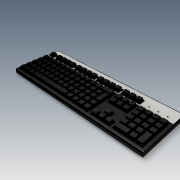
# Autodesk Inventor part: Teclado HP
Saved by Autodesk Inventor 2017 SP1 (Build 210196100, 196)
## iProperties
Created: 2013-08-30
Part Number: Teclado HP
Material: Generic
Document SubType Name: Modeling
Designer: MARCELO
Density: 1 g/cm^3
Mass: 1343.46 g
Surface Area: 2506.42 cm^2
Volume: 1343.46 cm^3
Appearance: Low Gloss - Black
Author: MARCELO
Autodesk Inventor part; units mm, degrees
ref_plane "YZ Plane" through (0, 0, 0) normal (1, 0, 0) x (0, 1, 0)
ref_plane "XZ Plane" through (0, 0, 0) normal (0, 1, 0) x (-1, 0, 0)
ref_plane "XY Plane" through (0, 0, 0) normal (0, 0, 1) x (1, 0, 0)
sketch "Sketch1" plane through (0, 0, 0) normal (0, 1, 0) x (-1, 0, 0)
  line L0 (0, 0) -> (-450, 0)
  line L1 (-450, 0) -> (-450, -160)
  line L2 (-450, -160) -> (0, -160)
  line L3 (0, -160) -> (0, 0)
  dimension "d0" = 450
  dimension "d2" = 160
  constraints: 8 end point, 2 parallel, 1 horizontal, 1 perpendicular
  measures "d0" distance between parallel lines of L1 L3
  measures "d2" distance between parallel lines of L2 L0
extrude "Extrusion1" add sketch "Sketch1" along normal blind 17
fillet "Fillet1" radius 10 2 edges at (450, 8.5, -160) (0, 8.5, -160)
fillet "Fillet1" radius 5 2 edges at (225, 17, 0) (225, 0, 0)
sketch "Sketch2" plane through (0, 17, 0) normal (0, 1, 0) x (1, 0, 0)
  line L0 (450, 5) -> (0, 5) projected
  line L1 (450, 5) -> (450, 150) projected
  line L2 (0, 150) -> (0, 5) projected
  line L3 (6, 9) -> (288, 9)
  line L4 (288, 111) -> (6, 111)
  line L5 (6, 111) -> (6, 9)
  line L6 (293, 31) -> (313, 31)
  line L7 (313, 31) -> (313, 51)
  line L8 (313, 51) -> (335, 51)
  line L9 (335, 51) -> (335, 31)
  line L10 (335, 31) -> (355, 31)
  line L11 (355, 31) -> (355, 9)
  line L12 (355, 9) -> (293, 9)
  line L13 (360, 9) -> (442, 9)
  line L14 (442, 9) -> (442, 111)
  line L15 (442, 111) -> (360, 111)
  line L16 (360, 111) -> (360, 9)
  line L17 (6, 117) -> (28, 117)
  line L18 (28, 117) -> (28, 139)
  line L19 (28, 139) -> (6, 139)
  line L20 (6, 139) -> (6, 117)
  line L21 (289, 117) -> (207, 117)
  line L22 (207, 117) -> (207, 139)
  line L23 (207, 139) -> (289, 139)
  line L24 (289, 139) -> (289, 117)
  line L25 (203, 117) -> (121, 117)
  line L26 (121, 117) -> (121, 139)
  line L27 (121, 139) -> (203, 139)
  line L28 (203, 139) -> (203, 117)
  line L29 (35, 139) -> (117, 139)
  line L30 (117, 139) -> (117, 117)
  line L31 (117, 117) -> (35, 117)
  line L32 (35, 117) -> (35, 139)
  line L33 (293, 111) -> (355, 111)
  line L34 (355, 111) -> (355, 69)
  line L35 (355, 69) -> (293, 69)
  line L36 (293, 117) -> (355, 117)
  line L37 (355, 117) -> (355, 139)
  line L38 (355, 139) -> (293, 139)
  line L39 (293, 139) -> (293, 117)
  circle A0 centre (376, 126) radius 2
  circle A1 centre (401, 126) radius 2
  circle A2 centre (426, 126) radius 2
  line L40 (401, 126) -> (401, 111) construction
  line L41 (288, 111) -> (288, 9)
  line L42 (440, 160) -> (10, 160) projected
  line L43 (293, 31) -> (293, 9)
  line L44 (293, 69) -> (293, 111)
  point P0 (0, 0)
  dimension "d7" = 6
  dimension "d9" = 4
  dimension "d10" = 102
  dimension "d12" = 22
  dimension "d13" = 20
  dimension "d15" = 22
  dimension "d17" = 82
  dimension "d18" = 5
  dimension "d19" = 22
  dimension "d20" = 6
  dimension "d21" = 22
  dimension "d22" = 82
  dimension "d24" = 82
  dimension "d26" = 82
  dimension "d27" = 42
  dimension "d28" = 4
  dimension "d29" = 50
  dimension "d30" = 15
  dimension "d87" = 4
  dimension "d88" = 4
  dimension "d89" = 282
  dimension "d90" = 5
  dimension "d91" = 20
  dimension "d92" = 62
  dimension "d163" = 62
  dimension "d164" = 4
  constraints: 82 end point, 19 collinear, 17 parallel, 9 perpendicular, 8 horizontal, 3 centre point, 2 equal radius, 1 horizontal alignment, 1 midpoint, 1 symmetric about line
  measures "d7" distance between parallel lines of L5 L2
  measures "d9" distance between parallel lines of L0 L3
  measures "d10" distance between parallel lines of L3 L4
  measures "d12" distance between parallel lines of L12 L6
  measures "d13" distance between parallel lines of L8 L6
  measures "d15" distance between parallel lines of L9 L7
  measures "d17" distance between parallel lines of L14 L16
  measures "d18" distance between parallel lines of L16 L11
  measures "d19" distance between parallel lines of L18 L20
  measures "d20" distance between parallel lines of L4 L17
  measures "d21" distance between parallel lines of L19 L17
  measures "d22" distance between parallel lines of L24 L22
  measures "d24" distance between parallel lines of L28 L26
  measures "d26" distance between parallel lines of L30 L32
  measures "d27" distance between parallel lines of L35 L33
  measures "d28" diameter of A1
  measures "d29" distance of A2.centre A0.centre
  measures "d30" distance of L40.start L40.end
  measures "d87" distance between parallel lines of L22 L28
  measures "d88" distance between parallel lines of L26 L30
  measures "d89" distance between parallel lines of L41 L5
  measures "d90" distance between parallel lines of L43 L41
  measures "d91" distance between parallel lines of L7 L43
  measures "d92" distance between parallel lines of L11 L43
  measures "d163" distance between parallel lines of L37 L39
  measures "d164" distance between parallel lines of L39 L24
extrude "Extrusion2" cut sketch "Sketch2" against normal blind 5
sketch "Sketch3" plane through (0, 12, 0) normal (0, 1, 0) x (1, 0, 0)
  line L0 (28, 117) -> (6, 117) projected
  line L1 (28, 139) -> (28, 117) projected
  line L2 (6, 139) -> (28, 139) projected
  line L3 (6, 117) -> (6, 139) projected
  line L4 (35, 139) -> (117, 139) projected
  line L5 (35, 117) -> (35, 139) projected
  line L6 (117, 117) -> (35, 117) projected
  line L7 (117, 139) -> (117, 117) projected
  line L8 (203, 117) -> (121, 117) projected
  line L9 (203, 139) -> (203, 117) projected
  line L10 (121, 139) -> (203, 139) projected
  line L11 (121, 117) -> (121, 139) projected
  line L12 (289, 117) -> (207, 117) projected
  line L13 (289, 139) -> (289, 117) projected
  line L14 (207, 139) -> (289, 139) projected
  line L15 (207, 117) -> (207, 139) projected
  line L16 (355, 117) -> (293, 117) projected
  line L17 (355, 139) -> (355, 117) projected
  line L18 (293, 139) -> (355, 139) projected
  line L19 (293, 117) -> (293, 139) projected
  line L20 (293, 111) -> (355, 111) projected
  line L21 (355, 69) -> (293, 69) projected
  line L22 (355, 111) -> (355, 69) projected
  line L23 (355, 9) -> (293, 9) projected
  line L24 (355, 31) -> (355, 9) projected
  line L25 (335, 31) -> (355, 31) projected
  line L26 (335, 51) -> (335, 31) projected
  line L27 (313, 51) -> (335, 51) projected
  line L28 (313, 31) -> (313, 51) projected
  line L29 (293, 31) -> (313, 31) projected
  line L30 (442, 9) -> (360, 9) projected
  line L31 (442, 111) -> (442, 9) projected
  line L32 (360, 111) -> (442, 111) projected
  line L33 (360, 9) -> (360, 111) projected
  line L34 (26, 137) -> (26, 119)
  line L35 (26, 119) -> (8, 119)
  line L36 (8, 119) -> (8, 137)
  line L37 (8, 137) -> (26, 137)
  line L38 (37, 137) -> (55, 137)
  line L39 (55, 137) -> (55, 119)
  line L40 (55, 119) -> (37, 119)
  line L41 (37, 119) -> (37, 137)
  line L42 (57, 137) -> (75, 137)
  line L43 (75, 137) -> (75, 119)
  line L44 (75, 119) -> (57, 119)
  line L45 (57, 119) -> (57, 137)
  line L46 (77, 137) -> (95, 137)
  line L47 (95, 137) -> (95, 119)
  line L48 (95, 119) -> (77, 119)
  line L49 (77, 119) -> (77, 137)
  line L50 (97, 137) -> (115, 137)
  line L51 (115, 137) -> (115, 119)
  line L52 (115, 119) -> (97, 119)
  line L53 (97, 119) -> (97, 137)
  line L54 (117, 117) -> (121, 117) construction
  line L55 (119, 117) -> (119, 144) construction
  line L56 (201, 137) -> (183, 137)
  line L57 (183, 137) -> (183, 119)
  line L58 (183, 119) -> (201, 119)
  line L59 (201, 119) -> (201, 137)
  line L60 (181, 137) -> (163, 137)
  line L61 (163, 137) -> (163, 119)
  line L62 (163, 119) -> (181, 119)
  line L63 (181, 119) -> (181, 137)
  line L64 (161, 137) -> (143, 137)
  line L65 (143, 137) -> (143, 119)
  line L66 (143, 119) -> (161, 119)
  line L67 (161, 119) -> (161, 137)
  line L68 (141, 137) -> (123, 137)
  line L69 (123, 137) -> (123, 119)
  line L70 (123, 119) -> (141, 119)
  line L71 (141, 119) -> (141, 137)
  line L72 (162, 139) -> (162, 117) construction
  line L73 (287, 137) -> (269, 137)
  line L74 (269, 137) -> (269, 119)
  line L75 (269, 119) -> (287, 119)
  line L76 (287, 119) -> (287, 137)
  line L77 (267, 137) -> (249, 137)
  line L78 (249, 137) -> (249, 119)
  line L79 (249, 119) -> (267, 119)
  line L80 (267, 119) -> (267, 137)
  line L81 (247, 137) -> (229, 137)
  line L82 (229, 137) -> (229, 119)
  line L83 (229, 119) -> (247, 119)
  line L84 (247, 119) -> (247, 137)
  line L85 (227, 137) -> (209, 137)
  line L86 (209, 137) -> (209, 119)
  line L87 (209, 119) -> (227, 119)
  line L88 (227, 119) -> (227, 137)
  line L89 (295, 137) -> (313, 137)
  line L90 (313, 137) -> (313, 119)
  line L91 (313, 119) -> (295, 119)
  line L92 (295, 119) -> (295, 137)
  line L93 (315, 137) -> (333, 137)
  line L94 (333, 137) -> (333, 119)
  line L95 (333, 119) -> (315, 119)
  line L96 (315, 119) -> (315, 137)
  line L97 (335, 137) -> (353, 137)
  line L98 (353, 137) -> (353, 119)
  line L99 (353, 119) -> (335, 119)
  line L100 (335, 119) -> (335, 137)
  line L101 (295, 109) -> (313, 109)
  line L102 (313, 91) -> (295, 91)
  line L103 (295, 91) -> (295, 109)
  line L104 (315, 49) -> (333, 49)
  line L105 (333, 49) -> (333, 31)
  line L106 (333, 31) -> (315, 31)
  line L107 (315, 31) -> (315, 49)
  line L108 (295, 29) -> (313, 29)
  line L109 (313, 29) -> (313, 11)
  line L110 (313, 11) -> (295, 11)
  line L111 (295, 11) -> (295, 29)
  line L112 (315, 29) -> (333, 29)
  line L113 (333, 29) -> (333, 11)
  line L114 (333, 11) -> (315, 11)
  line L115 (315, 11) -> (315, 29)
  line L116 (335, 29) -> (353, 29)
  line L117 (353, 29) -> (353, 11)
  line L118 (353, 11) -> (335, 11)
  line L119 (335, 11) -> (335, 29)
  line L120 (293, 9) -> (293, 31) projected
  line L121 (293, 69) -> (293, 111) projected
  line L122 (360, 9) -> (360, 111) projected
  line L123 (313, 91) -> (313, 109)
  line L124 (315, 109) -> (333, 109)
  line L125 (333, 91) -> (315, 91)
  line L126 (315, 91) -> (315, 109)
  line L127 (333, 91) -> (333, 109)
  line L128 (335, 109) -> (353, 109)
  line L129 (353, 91) -> (335, 91)
  line L130 (335, 91) -> (335, 109)
  line L131 (353, 91) -> (353, 109)
  line L132 (295, 89) -> (313, 89)
  line L133 (313, 71) -> (295, 71)
  line L134 (295, 71) -> (295, 89)
  line L135 (313, 71) -> (313, 89)
  line L136 (315, 89) -> (333, 89)
  line L137 (333, 71) -> (315, 71)
  line L138 (315, 71) -> (315, 89)
  line L139 (333, 71) -> (333, 89)
  line L140 (335, 89) -> (353, 89)
  line L141 (353, 71) -> (335, 71)
  line L142 (335, 71) -> (335, 89)
  line L143 (353, 71) -> (353, 89)
  line L144 (288, 9) -> (6, 9) projected
  line L145 (288, 111) -> (288, 9) projected
  line L146 (6, 111) -> (288, 111) projected
  line L147 (6, 9) -> (6, 111) projected
  point P0 (0, 0)
  dimension "d33" = 2
  dimension "d34" = 2
  dimension "d35" = 2
  dimension "d36" = 2
  dimension "d37" = 2
  dimension "d38" = 18
  dimension "d39" = 2
  dimension "d40" = 2
  dimension "d41" = 2
  dimension "d42" = 2
  dimension "d43" = 18
  dimension "d44" = 18
  dimension "d45" = 2
  dimension "d47" = 18
  dimension "d51" = 2
  dimension "d52" = 2
  dimension "d53" = 2
  dimension "d93" = 2
  dimension "d94" = 2
  dimension "d95" = 18
  dimension "d98" = 20
  dimension "d101" = 20
  dimension "d104" = 18
  dimension "d105" = 2
  dimension "d106" = 18
  dimension "d107" = 2
  dimension "d108" = 18
  dimension "d109" = 18
  constraints: 214 end point, 32 symmetric about line, 24 parallel, 23 collinear, 13 horizontal, 13 perpendicular, 3 midpoint, 1 vertical, 43 other
  measures "d33" distance between parallel lines of L37 L2
  measures "d34" distance between parallel lines of L41 L5
  measures "d35" distance between parallel lines of L45 L39
  measures "d36" distance between parallel lines of L49 L43
  measures "d37" distance between parallel lines of L53 L47
  measures "d38" distance of L38.start L38.end
  measures "d39" distance between parallel lines of L92 L19
  measures "d40" distance between parallel lines of L96 L90
  measures "d41" distance between parallel lines of L100 L94
  measures "d42" distance between parallel lines of L17 L98
  measures "d43" distance between parallel lines of L90 L92
  measures "d44" distance between parallel lines of L94 L96
  measures "d45" distance between parallel lines of L101 L20
  measures "d47" distance between parallel lines of L102 L101
  measures "d51" distance between parallel lines of L23 L110
  measures "d52" distance between parallel lines of L104 L27
  measures "d53" distance between parallel lines of L108 L29
  measures "d93" distance between parallel lines of L111 L120
  measures "d94" distance between parallel lines of L103 L121
  measures "d95" distance between parallel lines of L123 L103
  measures "d98" distance of L102.end L126.start
  measures "d101" distance of L102.end L134.start
  measures "d104" distance between parallel lines of L109 L111
  measures "d105" distance between parallel lines of L115 L109
  measures "d106" distance between parallel lines of L113 L115
  measures "d107" distance between parallel lines of L119 L113
  measures "d108" distance between parallel lines of L117 L119
  measures "d109" distance between parallel lines of L106 L104
sketch "Sketch5" plane through (0, 17, 0) normal (0, 1, 0) x (1, 0, 0)
  line L0 (35, 117) -> (35, 139) projected
  line L1 (35, 139) -> (117, 139) projected
  line L2 (117, 139) -> (117, 117) projected
  line L3 (117, 117) -> (35, 117) projected
  line L4 (289, 139) -> (289, 117) projected
  line L5 (289, 117) -> (207, 117) projected
  line L6 (207, 117) -> (207, 139) projected
  line L7 (207, 139) -> (289, 139) projected
  line L8 (355, 139) -> (355, 117) projected
  line L9 (355, 117) -> (293, 117) projected
  line L10 (293, 117) -> (293, 139) projected
  line L11 (293, 139) -> (355, 139) projected
  line L12 (28, 139) -> (28, 117) projected
  line L13 (28, 117) -> (6, 117) projected
  line L14 (6, 117) -> (6, 139) projected
  line L15 (6, 139) -> (28, 139) projected
  line L16 (203, 139) -> (203, 117) projected
  line L17 (203, 117) -> (121, 117) projected
  line L18 (121, 117) -> (121, 139) projected
  line L19 (121, 139) -> (203, 139) projected
  line L20 (6, 111) -> (288, 111) projected
  arc A0 (450, 150) -> (440, 160) centre (440, 150) ccw projected
  line L21 (440, 160) -> (10, 160) projected
  line L22 (10, 158) -> (440, 158)
  arc A1 (448, 150) -> (440, 158) centre (440, 150) ccw
  line L23 (448, 150) -> (448, 113)
  line L24 (448, 10) -> (2, 10)
  line L25 (2, 113) -> (2, 150)
  line L26 (2, 113) -> (448, 113)
  line L27 (450, 5) -> (450, 150) projected
  line L28 (0, 150) -> (0, 5) projected
  arc A2 (10, 158) -> (2, 150) centre (10, 150) ccw
  point P0 (0, 0)
  dimension "d132" = 2
  dimension "d133" = 2
  dimension "d136" = 2
  dimension "d137" = 2
  constraints: 10 end point, 4 point on circle, 2 centre point, 2 tangent, 1 parallel, 1 perpendicular, 1 other
  measures "d132" distance between parallel lines of L22 L21
  measures "d133" distance between parallel lines of L20 L26
  measures "d136" distance between parallel lines of L25 L28
  measures "d137" distance between parallel lines of L27 L23
extrude "Extrusion5" cut sketch "Sketch5" against normal blind 1
extrude "Extrusion6" add sketch "Sketch3" along normal blind 13 draft -10 contours L34 L35 L36 L37 | L38 L39 L40 L41 | L42 L43 L44 L45 | L46 L47 L48 L49 | L50 L51 L52 L53 | L59 L58 L57 L56 | L63 L62 L61 L60 | L67 L66 L65 L64 | L71 L70 L69 L68 | L76 L75 L74 L73 | L80 L79 L78 L77 | L84 L83 L82 L81 | L88 L87 L86 L85 | L89 L90 L91 L92 | L93 L94 L95 L96 | L97 L98 L99 L100 | L101 L123 L102 L103 | L104 L105 L106 L107 | L108 L109 L110 L111 | L112 L113 L114 L115 | L116 L117 L118 L119 | L124 L127 L125 L126 | L128 L131 L129 L130 | L132 L135 L133 L134 | L136 L139 L137 L138 | L140 L143 L141 L142
sketch "Sketch6" plane through (0, 12, 0) normal (0, 1, 0) x (1, 0, 0)
  line L0 (6, 111) -> (288, 111) projected
  line L1 (6, 9) -> (6, 111) projected
  line L2 (442, 9) -> (360, 9) projected
  line L3 (442, 111) -> (442, 9) projected
  line L4 (360, 111) -> (442, 111) projected
  line L5 (360, 9) -> (360, 111) projected
  line L6 (8, 109) -> (26, 109)
  line L7 (26, 109) -> (26, 91)
  line L8 (26, 91) -> (8, 91)
  line L9 (8, 91) -> (8, 109)
  line L10 (28, 109) -> (46, 109)
  line L11 (46, 109) -> (46, 91)
  line L12 (46, 91) -> (28, 91)
  line L13 (28, 91) -> (28, 109)
  line L14 (48, 109) -> (66, 109)
  line L15 (66, 109) -> (66, 91)
  line L16 (66, 91) -> (48, 91)
  line L17 (48, 91) -> (48, 109)
  line L18 (68, 109) -> (86, 109)
  line L19 (86, 109) -> (86, 91)
  line L20 (86, 91) -> (68, 91)
  line L21 (68, 91) -> (68, 109)
  line L22 (88, 109) -> (106, 109)
  line L23 (106, 109) -> (106, 91)
  line L24 (106, 91) -> (88, 91)
  line L25 (88, 91) -> (88, 109)
  line L26 (108, 109) -> (126, 109)
  line L27 (126, 109) -> (126, 91)
  line L28 (126, 91) -> (108, 91)
  line L29 (108, 91) -> (108, 109)
  line L30 (128, 109) -> (146, 109)
  line L31 (146, 109) -> (146, 91)
  line L32 (146, 91) -> (128, 91)
  line L33 (128, 91) -> (128, 109)
  line L34 (148, 109) -> (166, 109)
  line L35 (166, 109) -> (166, 91)
  line L36 (166, 91) -> (148, 91)
  line L37 (148, 91) -> (148, 109)
  line L38 (168, 109) -> (186, 109)
  line L39 (186, 109) -> (186, 91)
  line L40 (186, 91) -> (168, 91)
  line L41 (168, 91) -> (168, 109)
  line L42 (188, 109) -> (206, 109)
  line L43 (206, 109) -> (206, 91)
  line L44 (206, 91) -> (188, 91)
  line L45 (188, 91) -> (188, 109)
  line L46 (208, 109) -> (226, 109)
  line L47 (226, 109) -> (226, 91)
  line L48 (226, 91) -> (208, 91)
  line L49 (208, 91) -> (208, 109)
  line L50 (228, 109) -> (246, 109)
  line L51 (246, 109) -> (246, 91)
  line L52 (246, 91) -> (228, 91)
  line L53 (228, 91) -> (228, 109)
  line L54 (248, 91) -> (248, 109)
  line L55 (248, 109) -> (286, 109)
  line L56 (286, 109) -> (286, 91)
  line L57 (286, 91) -> (248, 91)
  line L58 (8, 89) -> (26, 89)
  line L59 (26, 89) -> (26, 71)
  line L60 (26, 71) -> (8, 71)
  line L61 (8, 71) -> (8, 89)
  line L62 (28, 89) -> (46, 89)
  line L63 (46, 89) -> (46, 71)
  line L64 (46, 71) -> (28, 71)
  line L65 (28, 71) -> (28, 89)
  line L66 (48, 89) -> (66, 89)
  line L67 (66, 89) -> (66, 71)
  line L68 (66, 71) -> (48, 71)
  line L69 (48, 71) -> (48, 89)
  line L70 (68, 89) -> (86, 89)
  line L71 (86, 89) -> (86, 71)
  line L72 (86, 71) -> (68, 71)
  line L73 (68, 71) -> (68, 89)
  line L74 (88, 89) -> (106, 89)
  line L75 (106, 89) -> (106, 71)
  line L76 (106, 71) -> (88, 71)
  line L77 (88, 71) -> (88, 89)
  line L78 (108, 89) -> (126, 89)
  line L79 (126, 89) -> (126, 71)
  line L80 (126, 71) -> (108, 71)
  line L81 (108, 71) -> (108, 89)
  line L82 (128, 89) -> (146, 89)
  line L83 (146, 89) -> (146, 71)
  line L84 (146, 71) -> (128, 71)
  line L85 (128, 71) -> (128, 89)
  line L86 (148, 89) -> (166, 89)
  line L87 (166, 89) -> (166, 71)
  line L88 (166, 71) -> (148, 71)
  line L89 (148, 71) -> (148, 89)
  line L90 (168, 89) -> (186, 89)
  line L91 (186, 89) -> (186, 71)
  line L92 (186, 71) -> (168, 71)
  line L93 (168, 71) -> (168, 89)
  line L94 (188, 89) -> (206, 89)
  line L95 (206, 89) -> (206, 71)
  line L96 (206, 71) -> (188, 71)
  line L97 (188, 71) -> (188, 89)
  line L98 (208, 89) -> (226, 89)
  line L99 (226, 89) -> (226, 71)
  line L100 (226, 71) -> (208, 71)
  line L101 (208, 71) -> (208, 89)
  line L102 (228, 89) -> (246, 89)
  line L103 (246, 89) -> (246, 71)
  line L104 (246, 71) -> (228, 71)
  line L105 (228, 71) -> (228, 89)
  line L106 (248, 89) -> (266, 89)
  line L107 (266, 89) -> (266, 71)
  line L108 (266, 71) -> (248, 71)
  line L109 (248, 71) -> (248, 89)
  line L110 (268, 89) -> (286, 89)
  line L111 (8, 69) -> (26, 69)
  line L112 (26, 69) -> (26, 51)
  line L113 (26, 51) -> (8, 51)
  line L114 (8, 51) -> (8, 69)
  line L115 (28, 69) -> (46, 69)
  line L116 (46, 69) -> (46, 51)
  line L117 (46, 51) -> (28, 51)
  line L118 (28, 51) -> (28, 69)
  line L119 (48, 69) -> (66, 69)
  line L120 (66, 69) -> (66, 51)
  line L121 (66, 51) -> (48, 51)
  line L122 (48, 51) -> (48, 69)
  line L123 (68, 69) -> (86, 69)
  line L124 (86, 69) -> (86, 51)
  line L125 (86, 51) -> (68, 51)
  line L126 (68, 51) -> (68, 69)
  line L127 (88, 69) -> (106, 69)
  line L128 (106, 69) -> (106, 51)
  line L129 (106, 51) -> (88, 51)
  line L130 (88, 51) -> (88, 69)
  line L131 (108, 69) -> (126, 69)
  line L132 (126, 69) -> (126, 51)
  line L133 (126, 51) -> (108, 51)
  line L134 (108, 51) -> (108, 69)
  line L135 (128, 69) -> (146, 69)
  line L136 (146, 69) -> (146, 51)
  line L137 (146, 51) -> (128, 51)
  line L138 (128, 51) -> (128, 69)
  line L139 (148, 69) -> (166, 69)
  line L140 (166, 69) -> (166, 51)
  line L141 (166, 51) -> (148, 51)
  line L142 (148, 51) -> (148, 69)
  line L143 (168, 69) -> (186, 69)
  line L144 (186, 69) -> (186, 51)
  line L145 (186, 51) -> (168, 51)
  line L146 (168, 51) -> (168, 69)
  line L147 (188, 69) -> (206, 69)
  line L148 (206, 69) -> (206, 51)
  line L149 (206, 51) -> (188, 51)
  line L150 (188, 51) -> (188, 69)
  line L151 (208, 69) -> (226, 69)
  line L152 (226, 69) -> (226, 51)
  line L153 (226, 51) -> (208, 51)
  line L154 (208, 51) -> (208, 69)
  line L155 (228, 69) -> (246, 69)
  line L156 (246, 69) -> (246, 51)
  line L157 (246, 51) -> (228, 51)
  line L158 (228, 51) -> (228, 69)
  line L159 (248, 69) -> (266, 69)
  line L160 (266, 69) -> (266, 51)
  line L161 (266, 51) -> (248, 51)
  line L162 (248, 51) -> (248, 69)
  line L163 (286, 89) -> (286, 51)
  line L164 (286, 51) -> (268, 51)
  line L165 (268, 51) -> (268, 89)
  line L166 (8, 49) -> (26, 49)
  line L167 (26, 49) -> (26, 31)
  line L168 (26, 31) -> (8, 31)
  line L169 (8, 31) -> (8, 49)
  line L170 (28, 49) -> (46, 49)
  line L171 (46, 49) -> (46, 31)
  line L172 (46, 31) -> (28, 31)
  line L173 (28, 31) -> (28, 49)
  line L174 (48, 49) -> (66, 49)
  line L175 (66, 49) -> (66, 31)
  line L176 (66, 31) -> (48, 31)
  line L177 (48, 31) -> (48, 49)
  line L178 (68, 49) -> (86, 49)
  line L179 (86, 49) -> (86, 31)
  line L180 (86, 31) -> (68, 31)
  line L181 (68, 31) -> (68, 49)
  line L182 (88, 49) -> (106, 49)
  line L183 (106, 49) -> (106, 31)
  line L184 (106, 31) -> (88, 31)
  line L185 (88, 31) -> (88, 49)
  line L186 (108, 49) -> (126, 49)
  line L187 (126, 49) -> (126, 31)
  line L188 (126, 31) -> (108, 31)
  line L189 (108, 31) -> (108, 49)
  line L190 (128, 49) -> (146, 49)
  line L191 (146, 49) -> (146, 31)
  line L192 (146, 31) -> (128, 31)
  line L193 (128, 31) -> (128, 49)
  line L194 (148, 49) -> (166, 49)
  line L195 (166, 49) -> (166, 31)
  line L196 (166, 31) -> (148, 31)
  line L197 (148, 31) -> (148, 49)
  line L198 (168, 49) -> (186, 49)
  line L199 (186, 49) -> (186, 31)
  line L200 (186, 31) -> (168, 31)
  line L201 (168, 31) -> (168, 49)
  line L202 (188, 49) -> (206, 49)
  line L203 (206, 49) -> (206, 31)
  line L204 (206, 31) -> (188, 31)
  line L205 (188, 31) -> (188, 49)
  line L206 (208, 49) -> (226, 49)
  line L207 (226, 49) -> (226, 31)
  line L208 (226, 31) -> (208, 31)
  line L209 (208, 31) -> (208, 49)
  line L210 (228, 49) -> (246, 49)
  line L211 (246, 49) -> (246, 31)
  line L212 (246, 31) -> (228, 31)
  line L213 (228, 31) -> (228, 49)
  line L214 (248, 49) -> (266, 49)
  line L215 (266, 49) -> (266, 31)
  line L216 (266, 31) -> (248, 31)
  line L217 (248, 31) -> (248, 49)
  line L218 (268, 49) -> (286, 49)
  line L219 (286, 49) -> (286, 31)
  line L220 (286, 31) -> (268, 31)
  line L221 (268, 31) -> (268, 49)
  line L222 (8, 29) -> (26, 29)
  line L223 (26, 29) -> (26, 11)
  line L224 (26, 11) -> (8, 11)
  line L225 (8, 11) -> (8, 29)
  line L226 (28, 29) -> (46, 29)
  line L227 (46, 29) -> (46, 11)
  line L228 (46, 11) -> (28, 11)
  line L229 (28, 11) -> (28, 29)
  line L230 (48, 29) -> (66, 29)
  line L231 (66, 29) -> (66, 11)
  line L232 (66, 11) -> (48, 11)
  line L233 (48, 11) -> (48, 29)
  line L234 (68, 29) -> (206, 29)
  line L235 (206, 11) -> (68, 11)
  line L236 (68, 11) -> (68, 29)
  line L237 (206, 29) -> (206, 11)
  line L238 (208, 29) -> (226, 29)
  line L239 (226, 29) -> (226, 11)
  line L240 (226, 11) -> (208, 11)
  line L241 (208, 11) -> (208, 29)
  line L242 (228, 29) -> (246, 29)
  line L243 (246, 29) -> (246, 11)
  line L244 (246, 11) -> (228, 11)
  line L245 (228, 11) -> (228, 29)
  line L246 (248, 29) -> (266, 29)
  line L247 (266, 29) -> (266, 11)
  line L248 (266, 11) -> (248, 11)
  line L249 (248, 11) -> (248, 29)
  line L250 (268, 29) -> (286, 29)
  line L251 (286, 29) -> (286, 11)
  line L252 (286, 11) -> (268, 11)
  line L253 (268, 11) -> (268, 29)
  line L254 (362, 109) -> (380, 109)
  line L255 (380, 109) -> (380, 91)
  line L256 (380, 91) -> (362, 91)
  line L257 (362, 91) -> (362, 109)
  line L258 (382, 109) -> (400, 109)
  line L259 (400, 109) -> (400, 91)
  line L260 (400, 91) -> (382, 91)
  line L261 (382, 91) -> (382, 109)
  line L262 (402, 109) -> (420, 109)
  line L263 (420, 109) -> (420, 91)
  line L264 (420, 91) -> (402, 91)
  line L265 (402, 91) -> (402, 109)
  line L266 (422, 109) -> (440, 109)
  line L267 (440, 109) -> (440, 91)
  line L268 (440, 91) -> (422, 91)
  line L269 (422, 91) -> (422, 109)
  line L270 (362, 89) -> (380, 89)
  line L271 (380, 89) -> (380, 71)
  line L272 (380, 71) -> (362, 71)
  line L273 (362, 71) -> (362, 89)
  line L274 (382, 89) -> (400, 89)
  line L275 (400, 89) -> (400, 71)
  line L276 (400, 71) -> (382, 71)
  line L277 (382, 71) -> (382, 89)
  line L278 (402, 89) -> (420, 89)
  line L279 (420, 89) -> (420, 71)
  line L280 (420, 71) -> (402, 71)
  line L281 (402, 71) -> (402, 89)
  line L282 (422, 89) -> (440, 89)
  line L283 (440, 89) -> (440, 71)
  line L284 (440, 71) -> (422, 71)
  line L285 (422, 71) -> (422, 89)
  line L286 (362, 69) -> (380, 69)
  line L287 (380, 69) -> (380, 51)
  line L288 (380, 51) -> (362, 51)
  line L289 (362, 51) -> (362, 69)
  line L290 (382, 69) -> (400, 69)
  line L291 (400, 69) -> (400, 51)
  line L292 (400, 51) -> (382, 51)
  line L293 (382, 51) -> (382, 69)
  line L294 (402, 69) -> (420, 69)
  line L295 (420, 69) -> (420, 51)
  line L296 (420, 51) -> (402, 51)
  line L297 (402, 51) -> (402, 69)
  line L298 (422, 69) -> (440, 69)
  line L299 (440, 69) -> (440, 51)
  line L300 (440, 51) -> (422, 51)
  line L301 (422, 51) -> (422, 69)
  line L302 (362, 49) -> (380, 49)
  line L303 (380, 49) -> (380, 31)
  line L304 (380, 31) -> (362, 31)
  line L305 (362, 31) -> (362, 49)
  line L306 (382, 49) -> (400, 49)
  line L307 (400, 49) -> (400, 31)
  line L308 (400, 31) -> (382, 31)
  line L309 (382, 31) -> (382, 49)
  line L310 (402, 49) -> (420, 49)
  line L311 (420, 49) -> (420, 31)
  line L312 (420, 31) -> (402, 31)
  line L313 (402, 31) -> (402, 49)
  line L314 (422, 49) -> (440, 49)
  line L315 (362, 29) -> (400, 29)
  line L316 (400, 11) -> (362, 11)
  line L317 (362, 11) -> (362, 29)
  line L318 (400, 29) -> (400, 11)
  line L319 (402, 29) -> (420, 29)
  line L320 (420, 29) -> (420, 11)
  line L321 (420, 11) -> (402, 11)
  line L322 (402, 11) -> (402, 29)
  line L323 (440, 49) -> (440, 11)
  line L324 (440, 11) -> (422, 11)
  line L325 (422, 11) -> (422, 49)
  point P0 (0, 0)
  dimension "d141" = 2
  dimension "d142" = 2
  dimension "d143" = 18
  dimension "d144" = 18
  dimension "d151" = 2
  dimension "d152" = 2
  dimension "d153" = 18
  dimension "d154" = 18
  constraints: 640 end point, 4 parallel, 2 horizontal, 2 perpendicular
  measures "d141" distance between parallel lines of L9 L1
  measures "d142" distance between parallel lines of L6 L0
  measures "d143" distance between parallel lines of L7 L9
  measures "d144" distance between parallel lines of L8 L6
  measures "d151" distance between parallel lines of L254 L4
  measures "d152" distance between parallel lines of L257 L5
  measures "d153" distance between parallel lines of L256 L254
  measures "d154" distance between parallel lines of L255 L257
extrude "Extrusion7" add sketch "Sketch6" along normal blind 13 draft -10 contours L6 L7 L8 L9 | L10 L11 L12 L13 | L14 L15 L16 L17 | L18 L19 L20 L21 | L22 L23 L24 L25 | L26 L27 L28 L29 | L30 L31 L32 L33 | L34 L35 L36 L37 | L38 L39 L40 L41 | L42 L43 L44 L45 | L46 L47 L48 L49 | L50 L51 L52 L53 | L54 L55 L56 L57 | L58 L59 L60 L61 | L62 L63 L64 L65 | L66 L67 L68 L69 | L70 L71 L72 L73 | L74 L75 L76 L77 | L78 L79 L80 L81 | L82 L83 L84 L85 | L86 L87 L88 L89 | L90 L91 L92 L93 | L94 L95 L96 L97 | L98 L99 L100 L101 | L102 L103 L104 L105 | L106 L107 L108 L109 | L110 L163 L164 L165 | L111 L112 L113 L114 | L115 L116 L117 L118 | L119 L120 L121 L122 | L123 L124 L125 L126 | L127 L128 L129 L130 | L131 L132 L133 L134 | L135 L136 L137 L138 | L139 L140 L141 L142 | L143 L144 L145 L146 | L147 L148 L149 L150 | L151 L152 L153 L154 | L155 L156 L157 L158 | L159 L160 L161 L162 | L166 L167 L168 L169 | L170 L171 L172 L173 | L174 L175 L176 L177 | L178 L179 L180 L181 | L182 L183 L184 L185 | L186 L187 L188 L189 | L190 L191 L192 L193 | L194 L195 L196 L197 | L198 L199 L200 L201 | L202 L203 L204 L205 | L206 L207 L208 L209 | L210 L211 L212 L213 | L214 L215 L216 L217 | L218 L219 L220 L221 | L222 L223 L224 L225 | L226 L227 L228 L229 | L230 L231 L232 L233 | L234 L237 L235 L236 | L238 L239 L240 L241 | L242 L243 L244 L245 | L246 L247 L248 L249 | L250 L251 L252 L253 | L254 L255 L256 L257 | L258 L259 L260 L261 | L262 L263 L264 L265 | L266 L267 L268 L269 | L270 L271 L272 L273 | L274 L275 L276 L277 | L278 L279 L280 L281 | L282 L283 L284 L285 | L286 L287 L288 L289 | L290 L291 L292 L293 | L294 L295 L296 L297 | L298 L299 L300 L301 | L302 L303 L304 L305 | L306 L307 L308 L309 | L310 L311 L312 L313 | L314 L323 L324 L325 | L315 L318 L316 L317 | L319 L320 L321 L322
fillet "Fillet2" radius 2 16 edges at (0, 15.5355, -1.4645) (0, 8.5, 0) (0, 1.4645, -1.4645) (0, 0, -77.5) (2.9289, 0, -157.0711) (225, 0, -160) (447.0711, 0, -157.0711) (450, 0, -77.5) (450, 1.4645, -1.4645) (450, 8.5, 0) (450, 15.5355, -1.4645) (450, 17, -77.5) (447.0711, 17, -157.0711) (225, 17, -160) (2.9289, 17, -157.0711) (0, 17, -77.5)
body "Solid1"
